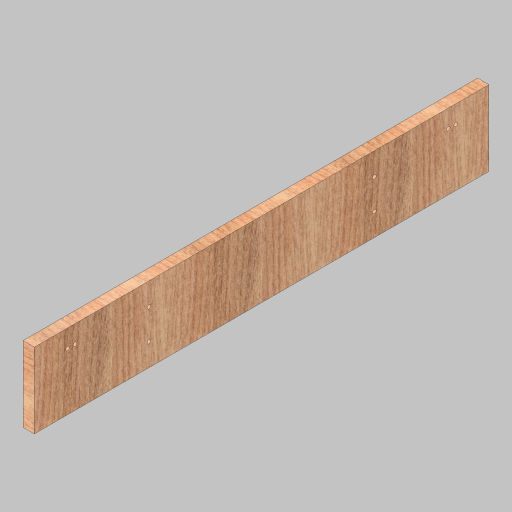
# Autodesk Inventor part: BP-001
Saved by Autodesk Inventor 2023.5 (Build 275446000, 446)
## iProperties
Created: 2025-01-26
Part Number: BP-001
Material: Wood (Birch)
Document SubType Name: Modeling
Designer: slick
Density: 0.55 g/cm^3
Appearance: Birch - Natural Polished
Author: slick
Autodesk Inventor part; units mm, degrees
ref_plane "YZ Plane" through (0, 0, 0) normal (1, 0, 0) x (0, 1, 0)
ref_plane "XZ Plane" through (0, 0, 0) normal (0, 1, 0) x (-1, 0, 0)
ref_plane "XY Plane" through (0, 0, 0) normal (0, 0, 1) x (1, 0, 0)
sketch "Sketch1" plane through (0, 0, 0) normal (1, 0, 0) x (0, 1, 0)
  line L0 (-63.5, -384.175) -> (63.5, -384.175)
  line L1 (63.5, -384.175) -> (63.5, 384.175)
  line L2 (63.5, 384.175) -> (-63.5, 384.175)
  line L3 (-63.5, 384.175) -> (-63.5, -384.175)
  line L4 (-63.5, -384.175) -> (63.5, 384.175) construction
  line L5 (63.5, -384.175) -> (-63.5, 384.175) construction
  point P0 (0, 0)
  dimension "d0" = 127
  dimension "d1" = 768.35
  constraints: 12 end point, 2 midpoint, 2 parallel, 1 horizontal, 1 perpendicular
  measures "d0" distance of L2.end L1.end
  measures "d1" distance of L0.end L1.end
extrude "Extrusion1" add sketch "Sketch1" along normal blind 19.05
sketch "Sketch2" plane through (19.05, 0, 0) normal (1, 0, 0) x (0, 0, -1)
  line L0 (-384.175, 63.5) -> (-384.175, -63.5) projected
  line L1 (384.175, 63.5) -> (-384.175, 63.5) construction
  line L2 (0, 63.5) -> (0, -63.5) construction
  line L3 (-384.175, -63.5) -> (384.175, -63.5) construction
  line L4 (-384.175, 63.5) -> (0, 63.5) construction
  line L5 (-190.5, 25.4) -> (-190.5, -25.4) construction
  point P0 (0, 0)
  point P1 (-328.0156, 33.3248)
  point P2 (-315.3156, 33.3248)
  point P3 (328.0156, 33.3248)
  point P4 (315.3156, 33.3248)
  point P5 (-192.0875, 63.5)
  point P6 (-190.5, 0)
  point P7 (0, 0)
  point P8 (190.5, 25.4)
  point P9 (190.5, -25.4)
  dimension "d4" = 12.7
  dimension "d5" = 56.1594
  dimension "d6" = 30.1752
  dimension "d14" = 50.8
  dimension "d16" = 193.675
  constraints: 6 end point, 5 midpoint, 4 symmetric about line, 2 horizontal alignment, 1 collinear, 1 vertical, 1 vertical alignment
  measures "d4" distance of point (-315.316, 33.325) point (-328.016, 33.325)
  measures "d5" distance from line of L0 point (-328.016, 33.325)
  measures "d6" distance from line of point (-328.016, 33.325) L1
  measures "d14" distance of L5.start L5.end
  measures "d16" distance from line of L0 L5.start
hole "Hole1" at (19.05, 33.3248, 328.0156) at (19.05, 33.3248, 315.3156) at (19.05, 33.3248, -315.3156) at (19.05, 33.3248, -328.0156) at (19.05, 25.4, 190.5) at (19.05, -25.4, 190.5) at (19.05, 25.4, -190.5) at (19.05, -25.4, -190.5) direction (-1, 0, 0) diameter 6.35 end through all
body "Solid1"
